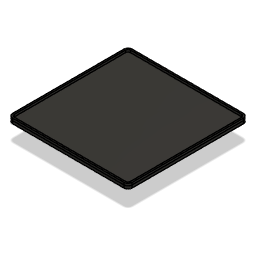
mouse pad base v1 (Autodesk Fusion 360 design; units mm, degrees)
Autodesk Fusion 360 part; units mm, degrees
sketch "Sketch1" plane through (0, 0, 0) normal (0, 1, 0) x (1, 0, 0)
  line L0 (-110, 110) -> (110, 110)
  line L1 (110, 110) -> (110, -110)
  line L2 (110, -110) -> (-110, -110)
  line L3 (-110, -110) -> (-110, 110)
  line L4 (-110, 110) -> (110, -110) construction
  line L5 (110, 110) -> (-110, -110) construction
  line L6 (107, -107) -> (-107, -107)
  line L7 (-107, -107) -> (-107, 107)
  line L8 (-107, 107) -> (107, 107)
  line L9 (107, 107) -> (107, -107)
  dimension "d1" = 220
  dimension "d2" = 220
  dimension "d3" = 3
  constraint horizontal L0
  constraint perpendicular L0 L1
  constraint parallel L0 L2
  constraint parallel L1 L3
  constraint coincident L4 origin
  constraint coincident L5 origin
  measures "d1" distance of L1.end L2.end
  measures "d2" distance of L0.end L1.end
extrude "Extrude1" add sketch "Sketch1" against normal blind 5 contours L0 L1 L2 L3 | L6 L7 L8 L9 makes body 1
extrude "Extrude2" add sketch "Sketch1" along normal blind 4 separate body makes body 2
sketch "Sketch2" plane through (0, -5, 0) normal (0, -1, 0) x (1, 0, 0)
  line L0 (110, 110) -> (-110, 110)
  line L1 (-110, 110) -> (-110, -110)
  line L2 (-110, -110) -> (110, -110)
  line L3 (110, -110) -> (110, 110)
  line L4 (-50, 30) -> (-50, -30)
  line L5 (-50, 30) -> (60, 30)
  line L6 (60, 30) -> (60, -30)
  line L7 (60, -30) -> (-50, -30)
  dimension "d8" = 60
  dimension "d11" = 30
  dimension "d12" = 60
  dimension "d13" = 110
  constraint vertical L4
  constraint perpendicular L4 L5
  constraint perpendicular L5 L6
  constraint perpendicular L4 L7
  measures "d8" distance of L4.start L4.end
  measures "d11" vertical distance of origin L4.start
  measures "d12" distance of L1 L4
  measures "d13" distance of L4.start L5.end
extrude "Extrude3" add sketch "Sketch2" along normal blind 30 contours L4 L5 L6 L7 bodies 2 1
chamfer "Chamfer1" distance 90 distance2 25 1 edges at (60, -35, 0) measured on face at (-13.3333, -35, 10) on bodies 1
sketch "Sketch3" plane through (-50, 0, 0) normal (-1, 0, 0) x (0, 0, 1)
  line L0 (30, -5) -> (-30, -5)
  line L1 (-30, -5) -> (-30, -35)
  line L2 (-30, -35) -> (30, -35)
  line L3 (30, -35) -> (30, -5)
  line L4 (0, -35) -> (-30, -5) construction
  line L5 (0, -35) -> (30, -5) construction
  circle A0 centre (-15, -20) radius 5
  circle A1 centre (-15, -20) radius 2.7
  circle A2 centre (15, -20) radius 5
  circle A3 centre (15, -20) radius 2.7
  dimension "d18" = 10
  dimension "d19" = 5.4
  constraint midpoint L2 L4.start
  constraint coincident L0.end L1.start
  constraint coincident L0.start L3.end
  constraint midpoint L4 A0.centre
  constraint concentric A0 A1
  constraint midpoint L5 A2.centre
  constraint concentric A2 A3
  constraint equal A1 A3
  constraint equal A0 A2
  measures "d18" diameter of A0
  measures "d19" diameter of A1
extrude "Extrude4" cut sketch "Sketch3" against normal blind 115 contours A0 | A1 | A2 | A3 bodies 1 2
extrude "Extrude5" add sketch "Sketch3" against normal blind 7 contours A0 | A2 bodies 1 2
fillet "Fillet1" radius 7.5 8 edges at (-110, -2.5, 110) (-110, 2, 110) (110, -2.5, 110) (110, 2, 110) (110, -2.5, -110) (110, 2, -110) (-110, -2.5, -110) (-110, 2, -110) on bodies 1 2
fillet "Fillet1" radius 4.5 4 edges at (-107, 2, -107) (-107, 2, 107) (107, 2, 107) (107, 2, -107) on bodies 1 2
chamfer "Chamfer2" distance 1 distance2 1 2 edges at (42, -15, 15) (42, -15, -15) measured on face at (-17.9483, -31.6523, 4.7818) measured on face at (-17.9483, -31.6523, 4.7818) on bodies 1
chamfer "Chamfer2" distance 0.4 distance2 0.4 2 faces at (-45.3333, -20.2688, -12.3134) (-45.3333, -20.2688, 17.6866) on bodies 1
copy_body "Body->Comp1" bodies 1 removing the originals makes body 3 in component "mouse pad base"
copy_body "Body->Comp2" bodies 2 removing the originals makes body 4 in component "mouse pad ridge"
component "mouse pad base" placed x (1, 0, 0) y (0, 1, 0) z (0, 0, 1) at (0, 0, 0)
component "mouse pad ridge" placed x (1, 0, 0) y (0, 1, 0) z (0, 0, 1) at (0, 0, 0)
named bodies: "mouse pad base", "mouse pad ridge"
